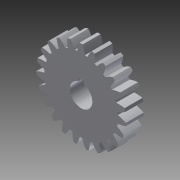
# Autodesk Inventor part: Gear for Angle
Saved by Autodesk Inventor 2014 SP1 (Build 180222100, 222)
## iProperties
Created: 2013-02-02
Part Number: Gear for Angle
Material: Aluminum 6061
Document SubType Name: Modeling
Designer: actoennies
Mass: 10.6641 g
Surface Area: 25.8868 cm^2
Volume: 3.9351 cm^3
Density: 2.71 g/cm^3
Appearance: Aluminum - Flat
Author: actoennies
Autodesk Inventor part; units mm, degrees
ref_plane "YZ Plane" through (0, 0, 0) normal (1, 0, 0) x (0, 1, 0)
ref_plane "XZ Plane" through (0, 0, 0) normal (0, 1, 0) x (-1, 0, 0)
ref_plane "XY Plane" through (0, 0, 0) normal (0, 0, 1) x (1, 0, 0)
sketch "Sketch1" plane through (0, 0, 0) normal (0, 0, 1) x (1, 0, 0)
  arc A0 (-4.8264, 15.2068) -> (-4.8046, 12.1837) centre (6.3519, 13.7758) ccw
  arc A1 (-4.8046, 12.1837) -> (-5.6249, 11.8275) centre (0, 0) ccw
  arc A2 (-5.6249, 11.8275) -> (-7.8194, 13.9068) centre (-14.4033, 4.7605) ccw
  arc A3 (-7.8194, 13.9068) -> (-8.7502, 13.3408) centre (0, 0) ccw
  arc A4 (-8.7502, 13.3408) -> (-7.9136, 10.4357) centre (2.3997, 14.9786) ccw
  arc A5 (-7.9136, 10.4357) -> (-8.6073, 9.8713) centre (0, 0) ccw
  arc A6 (-8.6073, 9.8713) -> (-11.2814, 11.2814) centre (-15.1536, 0.698) ccw
  arc A7 (-11.2814, 11.2814) -> (-12.025, 10.4853) centre (0, 0) ccw
  arc A8 (-12.025, 10.4853) -> (-10.4357, 7.9136) centre (-1.7305, 15.0706) ccw
  arc A9 (-10.4357, 7.9136) -> (-10.9514, 7.183) centre (0, 0) ccw
  arc A10 (-10.9514, 7.183) -> (-13.9068, 7.8194) centre (-14.78, -3.4163) ccw
  arc A11 (-13.9068, 7.8194) -> (-14.408, 6.8521) centre (0, 0) ccw
  arc A12 (-14.408, 6.8521) -> (-12.1837, 4.8046) centre (-5.7323, 14.0449) ccw
  arc A13 (-12.1837, 4.8046) -> (-12.4832, 3.962) centre (0, 0) ccw
  arc A14 (-12.4832, 3.962) -> (-15.5007, 3.7774) centre (-13.3102, -7.2772) ccw
  arc A15 (-15.5007, 3.7774) -> (-15.7224, 2.7108) centre (0, 0) ccw
  arc A16 (-15.7224, 2.7108) -> (-13.0282, 1.3393) centre (-9.309, 11.9775) ccw
  arc A17 (-13.0282, 1.3393) -> (-13.0892, 0.4471) centre (0, 0) ccw
  arc A18 (-13.0892, 0.4471) -> (-15.9451, -0.5447) centre (-10.8532, -10.5984) ccw
  arc A19 (-15.9451, -0.5447) -> (-15.8707, -1.6316) centre (0, 0) ccw
  arc A20 (-15.8707, -1.6316) -> (-12.9064, -2.2253) centre (-12.1953, 9.0218) ccw
  arc A21 (-12.9064, -2.2253) -> (-12.7245, -3.1009) centre (0, 0) ccw
  arc A22 (-12.7245, -3.1009) -> (-15.2068, -4.8264) centre (-7.5914, -13.1335) ccw
  arc A23 (-15.2068, -4.8264) -> (-14.842, -5.8529) centre (0, 0) ccw
  arc A24 (-14.842, -5.8529) -> (-11.8275, -5.6249) centre (-14.1771, 5.397) ccw
  arc A25 (-11.8275, -5.6249) -> (-11.416, -6.4189) centre (0, 0) ccw
  arc A26 (-11.416, -6.4189) -> (-13.3408, -8.7502) centre (-3.7665, -14.6946) ccw
  arc A27 (-13.3408, -8.7502) -> (-12.7125, -9.6402) centre (0, 0) ccw
  arc A28 (-12.7125, -9.6402) -> (-9.8713, -8.6073) centre (-15.1075, 1.3719) ccw
  arc A29 (-9.8713, -8.6073) -> (-9.2609, -9.2609) centre (0, 0) ccw
  arc A30 (-9.2609, -9.2609) -> (-10.4853, -12.025) centre (0.3377, -15.1659) ccw
  arc A31 (-10.4853, -12.025) -> (-9.6402, -12.7125) centre (0, 0) ccw
  arc A32 (-9.6402, -12.7125) -> (-7.183, -10.9514) centre (-14.9174, -2.7549) ccw
  arc A33 (-7.183, -10.9514) -> (-6.4189, -11.416) centre (0, 0) ccw
  arc A34 (-6.4189, -11.416) -> (-6.8521, -14.408) centre (4.4169, -14.5124) ccw
  arc A35 (-6.8521, -14.408) -> (-5.8529, -14.842) centre (0, 0) ccw
  arc A36 (-5.8529, -14.842) -> (-3.962, -12.4832) centre (-13.621, -6.6774) ccw
  arc A37 (-3.962, -12.4832) -> (-3.1009, -12.7245) centre (0, 0) ccw
  arc A38 (-3.1009, -12.7245) -> (-2.7108, -15.7224) centre (8.1685, -12.7825) ccw
  arc A39 (-2.7108, -15.7224) -> (-1.6316, -15.8707) centre (0, 0) ccw
  arc A40 (-1.6316, -15.8707) -> (-0.4471, -13.0892) centre (-11.3143, -10.1047) ccw
  arc A41 (-0.4471, -13.0892) -> (0.4471, -13.0892) centre (0, 0) ccw
  arc A42 (0.4471, -13.0892) -> (1.6316, -15.8707) centre (11.3143, -10.1047) ccw
  arc A43 (1.6316, -15.8707) -> (2.7108, -15.7224) centre (0, 0) ccw
  arc A44 (2.7108, -15.7224) -> (3.1009, -12.7245) centre (-8.1685, -12.7825) ccw
  arc A45 (3.1009, -12.7245) -> (3.962, -12.4832) centre (0, 0) ccw
  arc A46 (3.962, -12.4832) -> (5.8529, -14.842) centre (13.621, -6.6774) ccw
  arc A47 (5.8529, -14.842) -> (6.8521, -14.408) centre (0, 0) ccw
  arc A48 (6.8521, -14.408) -> (6.4189, -11.416) centre (-4.4169, -14.5124) ccw
  arc A49 (6.4189, -11.416) -> (7.183, -10.9514) centre (0, 0) ccw
  arc A50 (7.183, -10.9514) -> (9.6402, -12.7125) centre (14.9174, -2.7549) ccw
  arc A51 (9.6402, -12.7125) -> (10.4853, -12.025) centre (0, 0) ccw
  arc A52 (10.4853, -12.025) -> (9.2609, -9.2609) centre (-0.3377, -15.1659) ccw
  arc A53 (9.2609, -9.2609) -> (9.8713, -8.6073) centre (0, 0) ccw
  arc A54 (9.8713, -8.6073) -> (12.7125, -9.6402) centre (15.1075, 1.3719) ccw
  arc A55 (12.7125, -9.6402) -> (13.3408, -8.7502) centre (0, 0) ccw
  arc A56 (13.3408, -8.7502) -> (11.416, -6.4189) centre (3.7665, -14.6946) ccw
  arc A57 (11.416, -6.4189) -> (11.8275, -5.6249) centre (0, 0) ccw
  arc A58 (11.8275, -5.6249) -> (14.842, -5.8529) centre (14.1771, 5.397) ccw
  arc A59 (14.842, -5.8529) -> (15.2068, -4.8264) centre (0, 0) ccw
  arc A60 (15.2068, -4.8264) -> (12.7245, -3.1009) centre (7.5914, -13.1335) ccw
  arc A61 (12.7245, -3.1009) -> (12.9064, -2.2253) centre (0, 0) ccw
  arc A62 (12.9064, -2.2253) -> (15.8707, -1.6316) centre (12.1953, 9.0218) ccw
  arc A63 (15.8707, -1.6316) -> (15.9451, -0.5447) centre (0, 0) ccw
  arc A64 (15.9451, -0.5447) -> (13.0892, 0.4471) centre (10.8532, -10.5984) ccw
  arc A65 (13.0892, 0.4471) -> (13.0282, 1.3393) centre (0, 0) ccw
  arc A66 (13.0282, 1.3393) -> (15.7224, 2.7108) centre (9.309, 11.9775) ccw
  arc A67 (15.7224, 2.7108) -> (15.5007, 3.7774) centre (0, 0) ccw
  arc A68 (15.5007, 3.7774) -> (12.4832, 3.962) centre (13.3102, -7.2772) ccw
  arc A69 (12.4832, 3.962) -> (12.1837, 4.8046) centre (0, 0) ccw
  arc A70 (12.1837, 4.8046) -> (14.408, 6.8521) centre (5.7323, 14.0449) ccw
  arc A71 (14.408, 6.8521) -> (13.9068, 7.8194) centre (0, 0) ccw
  arc A72 (13.9068, 7.8194) -> (10.9514, 7.183) centre (14.78, -3.4163) ccw
  arc A73 (10.9514, 7.183) -> (10.4357, 7.9136) centre (0, 0) ccw
  arc A74 (10.4357, 7.9136) -> (12.025, 10.4853) centre (1.7305, 15.0706) ccw
  arc A75 (12.025, 10.4853) -> (11.2814, 11.2814) centre (0, 0) ccw
  arc A76 (11.2814, 11.2814) -> (8.6073, 9.8713) centre (15.1536, 0.698) ccw
  arc A77 (8.6073, 9.8713) -> (7.9136, 10.4357) centre (0, 0) ccw
  arc A78 (7.9136, 10.4357) -> (8.7502, 13.3408) centre (-2.3997, 14.9786) ccw
  arc A79 (8.7502, 13.3408) -> (7.8194, 13.9068) centre (0, 0) ccw
  arc A80 (7.8194, 13.9068) -> (5.6249, 11.8275) centre (14.4033, 4.7605) ccw
  arc A81 (5.6249, 11.8275) -> (4.8046, 12.1837) centre (0, 0) ccw
  arc A82 (4.8046, 12.1837) -> (4.8264, 15.2068) centre (-6.3519, 13.7758) ccw
  arc A83 (4.8264, 15.2068) -> (3.7774, 15.5007) centre (0, 0) ccw
  arc A84 (3.7774, 15.5007) -> (2.2253, 12.9064) centre (12.5848, 8.4699) ccw
  arc A85 (2.2253, 12.9064) -> (1.3393, 13.0282) centre (0, 0) ccw
  arc A86 (1.3393, 13.0282) -> (0.5447, 15.9451) centre (-9.833, 11.5512) ccw
  arc A87 (0.5447, 15.9451) -> (-0.5447, 15.9451) centre (0, 0) ccw
  arc A88 (-0.5447, 15.9451) -> (-1.3393, 13.0282) centre (9.833, 11.5512) ccw
  arc A89 (-1.3393, 13.0282) -> (-2.2253, 12.9064) centre (0, 0) ccw
  arc A90 (-2.2253, 12.9064) -> (-3.7774, 15.5007) centre (-12.5848, 8.4699) ccw
  arc A91 (-3.7774, 15.5007) -> (-4.8264, 15.2068) centre (0, 0) ccw
  arc A92 (-1, 3.873) -> (1, 3.873) centre (0, 0) ccw
  line L0 (-1, 3.873) -> (-1, 5)
  line L1 (-1, 5) -> (1, 5)
  line L2 (1, 5) -> (1, 3.873)
  dimension "d0" = 8
  dimension "d1" = 1
  dimension "d2" = 1
  dimension "d3" = 1
  constraints: 186 point on circle, 93 centre point, 6 end point, 1 coincident, 1 horizontal, 1 parallel, 1 vertical, 277 other
  measures "d0" diameter of A92
  measures "d1" distance from line of point (0, 0) L2
  measures "d2" distance from line of point (0, 0) L0
  measures "d3" distance edge to line of A92 L1
extrude "Extrusion1" add sketch "Sketch1" along normal blind 6.35
body "Solid1"
